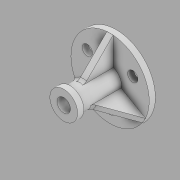
# Autodesk Inventor part: CStem A01209499
Saved by Autodesk Inventor 2020 (Build 240168000, 168)
## iProperties
Created: 2019-10-04
Part Number: CStem A01209499
Material: Genérico
Document SubType Name: Modeling
Designer: gerar
Density: 1 g/cm^3
Appearance: Valor por defecto
Author: gerar
Autodesk Inventor part; units mm, degrees
ref_plane "XZ Plane" through (0, 0, 0) normal (0, 1, 0) x (-1, 0, 0)
ref_plane "XY Plane" through (0, 0, 0) normal (0, 0, 1) x (1, 0, 0)
sketch "Boceto1" plane through (0, 0, 0) normal (0, 0, 1) x (1, 0, 0)
  circle A0 centre (0, 0) radius 76
  circle A1 centre (0, 0) radius 51 construction
  line L0 (0, 0) -> (54.9164, 31.706) construction
  line L1 (0, 0) -> (63.412, 0) construction
  circle A2 centre (44.1673, 25.5) radius 10
  circle A3 centre (-44.1673, 25.5) radius 10
  circle A4 centre (0, -51) radius 10
  dimension "d1" = 102
  dimension "d0" = 152
  dimension "d3" = 30
  dimension "d4" = 20
  dimension "d7" = 360
  constraints: 4 centre point, 4 coincident, 4 end point, 1 equal length, 1 horizontal, 1 point on line, 11 other
  measures "d0" diameter of A0
  measures "d3" angle of L1 L0
  measures "d4" diameter of A2
extrude "Extrusión1" add sketch "Boceto1" along normal blind 12
sketch "Boceto2" plane through (0, 0, 12) normal (0, 0, 1) x (1, 0, 0)
  circle A0 centre (0, 0) radius 22
  dimension "d11" = 44
  constraints: 1 centre point, 1 coincident
  measures "d11" diameter of A0
extrude "Extrusión2" add sketch "Boceto2" along normal blind 78
sketch "Boceto3" plane through (0, 0, 90) normal (0, 0, 1) x (1, 0, 0)
  circle A0 centre (0, 0) radius 27
  dimension "d14" = 54
  constraints: 1 centre point, 1 coincident
  measures "d14" diameter of A0
extrude "Extrusión3" add sketch "Boceto3" along normal blind 12
sketch "Boceto4" plane through (0, 0, 0) normal (1, 0, 0) x (0, 1, 0)
  line L0 (76, 12) -> (-76, 12) projected
  line L1 (76, 12) -> (22, 66)
  line L2 (22, 12) -> (22, 90) projected
  point P0 (0, 0)
  dimension "d17" = 45
  constraints: 2 end point, 1 point on line
  measures "d17" angle of L0 L1
extrude "Nervio1" add sketch "Boceto4" along normal mid plane 12 rib yes fills toward (0, 12.05) open curves L0 L1
ref_plane "Plano de trabajo2" through (0, 0, 0) normal (-0.5, 0.8660254, 0) x (0, 0, 1)
ref_plane "Plano de trabajo3" through (0, 0, 0) normal (0.5, 0.8660254, 0) x (0, 0, 1)
sketch "Boceto6" plane through (0, 0, 0) normal (-0.5, 0.8660254, 0) x (0, 0, 1)
  line L0 (12, -76) -> (12, 76) projected
  line L1 (12, -76) -> (66, -22)
  line L2 (12, -22) -> (90, -22) projected
  line L3 (12, -76) -> (88.3675, -76) construction
  point P0 (0, 0)
  point P1 (12, 32.6852)
  point P2 (12, 43.0775)
  dimension "d35" = 45
  constraints: 4 end point, 1 equal length, 1 horizontal, 1 point on line
  measures "d35" angle of L3 L1
extrude "Nervio3" add sketch "Boceto6" along normal mid plane 12 rib yes fills toward (12.05, 0) open curves L0 L1
sketch "Boceto7" plane through (0, 0, 0) normal (0.5, 0.8660254, 0) x (0, 0, 1)
  line L0 (12, -32.6852) -> (12, 76) projected
  line L1 (12, 76) -> (66.3426, 21.6574)
  line L2 (12, 76) -> (88.8521, 76) construction
  point P0 (0, 0)
  dimension "d42" = 45
  constraints: 4 end point, 1 equal length, 1 horizontal
  measures "d42" angle of L1 L2
extrude "Nervio4" add sketch "Boceto7" along normal mid plane 12 rib yes fills toward (12.05, 21.6574) open curves L0 L1
sketch "Boceto8" plane through (0, 0, 102) normal (0, 0, 1) x (1, 0, 0)
  point P0 (0, 0)
  point P1 (0, 0)
  constraints: 1 coincident
hole "Agujero1" at (0, 0, 102) direction (0, 0, -1) diameter 26 end through all
fillet "Empalme1" radius 10 3 edges at (0, 22, 66) (19.0526, -11, 66) (-19.0526, -11, 66)
